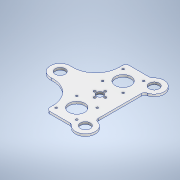
# Autodesk Inventor part: De_Tren
Saved by Autodesk Inventor 2022 (Build 260153000, 153)
## iProperties
Created: 2022-11-10
Part Number: De_Tren
Material: Aluminum 6061
Document SubType Name: Modeling
Designer: nguye
Density: 2.7 g/cm^3
Appearance: Aluminum - Flat
Author: nguye
Autodesk Inventor part; units mm, degrees
ref_plane "YZ Plane" through (0, 0, 0) normal (1, 0, 0) x (0, 1, 0)
ref_plane "XZ Plane" through (0, 0, 0) normal (0, 1, 0) x (-1, 0, 0)
ref_plane "XY Plane" through (0, 0, 0) normal (0, 0, 1) x (1, 0, 0)
sketch "Sketch1" plane through (0, 0, 0) normal (0, 1, 0) x (-1, 0, 0)
  circle A0 centre (0, 0) radius 60
  circle A1 centre (60, 0) radius 7.5
  circle A2 centre (-30, 51.9615) radius 7.5
  circle A3 centre (-30, -51.9615) radius 7.5
  circle A4 centre (0, -35) radius 12
  line L0 (0, -118.7756) -> (0, 118.7756) projected
  line L1 (121.2, 0) -> (-90.2, 0) projected
  circle A5 centre (0, 35) radius 12
  line L2 (21, 10) -> (-21, 10)
  line L3 (-21, 10) -> (-21, 60)
  line L4 (-21, 60) -> (21, 60)
  line L5 (21, 60) -> (21, 10)
  line L6 (21, 10) -> (-21, 60) construction
  line L7 (-21, 10) -> (21, 60) construction
  line L8 (21, -60) -> (-21, -60)
  line L9 (-21, -60) -> (-21, -10)
  line L10 (-21, -10) -> (21, -10)
  line L11 (21, -10) -> (21, -60)
  line L12 (21, -60) -> (-21, -10) construction
  line L13 (-21, -60) -> (21, -10) construction
  circle A6 centre (60, 0) radius 15
  circle A7 centre (-30, 51.9615) radius 15
  circle A8 centre (-30, -51.9615) radius 15
  circle A9 centre (56, 49.8397) radius 35
  circle A10 centre (56, -49.8397) radius 35
  circle A11 centre (0, 0) radius 5.15
  circle A12 centre (16, 55) radius 5
  circle A13 centre (16, -55) radius 5
  circle A14 centre (-14.8343, -65) radius 5
  circle A15 centre (-14.8343, 65) radius 5
  line L14 (-30, -36.9615) -> (-30, 36.9615)
  circle A16 centre (-35, -32.5966) radius 5
  circle A17 centre (-35, 32.5966) radius 5
  circle A18 centre (0, -8) radius 1.75
  circle A19 centre (8, 0) radius 1.75
  circle A20 centre (0, 8) radius 1.75
  circle A21 centre (-8, 0) radius 1.75
  line L15 (0, -9.75) -> (0, -10)
  point P0 (58.8, 14.9519)
  point P1 (21, 49.8397)
  point P2 (21, 55)
  point P3 (16, 60)
  point P4 (-16.174, 57.7789)
  point P5 (-21, 56.3204)
  point P6 (-21, -56.3204)
  point P7 (16, -60)
  point P8 (21, -55)
  point P9 (21, -49.8397)
  point P10 (58.8, -14.9519)
  point P11 (20.8372, -56.2655)
  point P12 (21, -56.205)
  point P13 (12.5965, -58.6628)
  point P14 (0, -60)
  point P15 (20.8372, 56.2655)
  point P16 (21, 56.205)
  point P17 (12.5965, 58.6628)
  point P18 (-21, -39.9615)
  point P19 (0, -10)
  point P20 (0, -5.15)
  point P21 (-5.15, 0)
  point P22 (-21, -56.205)
  point P23 (-16.174, -57.7789)
  point P24 (0, -60)
  point P25 (0, -47)
  point P26 (0, -23)
  point P27 (0, 5.15)
  point P28 (0, 10)
  point P29 (-21, 39.9615)
  point P30 (0, 60)
  point P31 (0, 23)
  point P32 (0, 47)
  point P33 (0, 60)
  point P34 (5.15, 0)
  point P35 (45, 0)
  point P36 (21.546, -55.9979)
  point P37 (58.1195, -14.904)
  point P38 (58.125, -14.8824)
  point P39 (58.1195, 14.904)
  point P40 (21.546, 55.9979)
  point P41 (58.125, 14.8824)
  point P42 (-60, 0)
  point P43 (-41.951, -42.8966)
  point P44 (-23.2831, -55.2982)
  point P45 (-36.2481, -47.8129)
  point P46 (-36.2481, 47.8129)
  point P47 (-23.2831, 55.2982)
  point P48 (-21, 56.205)
  point P49 (75, 0)
  point P50 (59.5312, 7.4853)
  point P51 (67.5, 0)
  point P52 (59.5312, -7.4853)
  point P53 (52.5, 0)
  point P54 (60, 0)
  point P55 (-41.951, 42.8966)
  point P56 (-17.3358, -60)
  point P57 (-17.3358, 60)
  point P58 (-14.8343, 60)
  point P59 (-18.6257, 61.7404)
  point P60 (-33.75, 37.4378)
  point P61 (-30, 32.5966)
  point P62 (-30, -32.5966)
  point P63 (-33.75, -37.4378)
  point P64 (-18.6257, -61.7404)
  point P65 (-14.8343, -60)
  point P66 (-30, 0)
  dimension "d0" = 120
  dimension "d13" = 30
  dimension "d14" = 30
  dimension "d28" = 3.5
  dimension "d1" = 15
  dimension "d4" = 360
  dimension "d6" = 24
  dimension "d7" = 35
  dimension "d8" = 42
  dimension "d9" = 50
  dimension "d10" = 42
  dimension "d11" = 50
  dimension "d12" = 30
  dimension "d15" = 70
  dimension "d16" = 10.3
  dimension "d19" = 10
  dimension "d20" = 10
  dimension "d23" = 10
  dimension "d24" = 10
  dimension "d25" = 30
  dimension "d26" = 10
  dimension "d27" = 10
  dimension "d29" = 8
  dimension "d32" = 360
  constraints: 28 end point, 18 centre point, 10 tangent, 5 coincident, 5 midpoint, 4 parallel, 2 horizontal, 2 perpendicular, 2 point on line, 2 symmetric about line, 2 vertical alignment, 1 horizontal alignment, 1 vertical, 33 other
  measures "d1" diameter of A1
  measures "d6" diameter of A4
  measures "d7" distance of point (0, 0) A5.centre
  measures "d8" distance of L3.end L4.end
  measures "d9" distance of L2.end L3.end
  measures "d10" distance of L9.end L10.end
  measures "d11" distance of L8.end L9.end
  measures "d12" diameter of A6
  measures "d15" diameter of A9
  measures "d16" diameter of A11
  measures "d19" diameter of A12
  measures "d20" diameter of A13
  measures "d23" diameter of A14
  measures "d24" diameter of A15
  measures "d25" distance from line of L14 point (0, 0)
  measures "d26" diameter of A16
  measures "d27" diameter of A17
  measures "d29" distance of point (0, 0) point (0, -8)
extrude "Extrusion1" add sketch "Sketch1" along normal blind 3.5 contours A1 L1 A6 A0 | A0 A6 L1 A1 | A1 L1 A6 A0 | A0 A6 L1 A1 | A6 L1 A19 A11 L0 A20 L2 L5 A9 A0 | A0 A10 L11 L10 L0 A18 A11 L1 A19 A6 | L5 L2 L0 A5 A0 A12 | L11 A13 A0 L0 A4 L10 | A12 A0 | A13 A0 | A0 A12 | A0 L4 A12 | L2 L3 A7 A0 L0 A5 | L0 A20 A11 L1 A21 L14 A7 L3 L2 | A13 A0 | L10 L9 A8 L14 L1 A21 A11 L0 A18 | L0 A4 A0 A8 L9 L10 | A13 L8 A0 | A0 A7 L4 | L8 A8 A0 | A7 L3 A0 | A0 L3 L4 A7 | L4 A7 A15 | A7 A0 A2 L3 | A8 A0 L9 | L9 A0 A3 A8 | A8 L8 L9 A0 | A14 A8 L8 | A0 A2 A7 L4 L3 | L14 A17 A7 | L9 L8 A8 A0 A3 | A8 A16 L14
sketch "Sketch2" plane through (0, 3.5, 0) normal (0, 1, 0) x (1, 0, 0)
  circle A0 centre (0, -35) radius 12 projected
  line L0 (-99, 0) -> (69, 0) projected
  point P0 (0, 0)
  point P1 (15.5, -50.5)
  point P2 (-15.5, -50.5)
  point P3 (-15.5, -19.5)
  point P4 (15.5, -19.5)
  point P5 (15.5, 50.5)
  point P6 (-15.5, 50.5)
  point P7 (-15.5, 19.5)
  point P8 (15.5, 19.5)
  dimension "d34" = 15.5
  dimension "d35" = 31
  dimension "d36" = 15.5
  dimension "d37" = 31
  constraints: 4 symmetric about line, 2 horizontal alignment, 2 vertical alignment
  measures "d34" horizontal distance of A0.centre point (-15.5, -50.5)
  measures "d35" distance of point (-15.5, -19.5) point (-15.5, -50.5)
  measures "d36" horizontal distance of A0.centre point (15.5, -50.5)
  measures "d37" distance of point (15.5, -50.5) point (-15.5, -50.5)
hole "Hole1" at (15.5, 3.5, 50.5) at (-15.5, 3.5, 50.5) at (-15.5, 3.5, 19.5) at (15.5, 3.5, 19.5) at (15.5, 3.5, -50.5) at (-15.5, 3.5, -50.5) at (-15.5, 3.5, -19.5) at (15.5, 3.5, -19.5) direction (0, -1, 0) diameter 3.05 end through all
body "Solid1"
